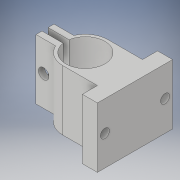
# Autodesk Inventor part: round_adaptor_13
Saved by Autodesk Inventor 2019 (Build 230136000, 136)
## iProperties
Created: 2018-09-01
Part Number: round_adaptor_13
Material: Generic
Document SubType Name: Modeling
Designer: cruiser
Density: 1 g/cm^3
Appearance: Default
Author: cruiser
Autodesk Inventor part; units mm, degrees
ref_plane "YZ Plane" through (0, 0, 0) normal (1, 0, 0) x (0, 1, 0)
ref_plane "XZ Plane" through (0, 0, 0) normal (0, 1, 0) x (-1, 0, 0)
ref_plane "XY Plane" through (0, 0, 0) normal (0, 0, 1) x (1, 0, 0)
sketch "Sketch1" plane through (0, 0, 0) normal (0, 1, 0) x (-1, 0, 0)
  arc A0 (0, 6.5) -> (0, -6.5) centre (0, 0) ccw
  arc A1 (7.433, 1) -> (6.8739, 3) centre (0, 0) ccw
  line L0 (0, 7.5) -> (-16.5, 7.5)
  line L1 (-16.5, 7.5) -> (-16.5, -7.5)
  line L2 (-16.5, -7.5) -> (0, -7.5)
  line L3 (0, -7.5) -> (0, -6.5)
  line L4 (-16.5, 12.5) -> (-11.5, 12.5)
  line L5 (-11.5, 12.5) -> (-11.5, 7.5)
  line L6 (-11.5, 7.5) -> (-16.5, 7.5)
  line L7 (-16.5, 7.5) -> (-16.5, 12.5)
  line L8 (-16.5, -7.5) -> (-11.5, -7.5)
  line L9 (-11.5, -7.5) -> (-11.5, -12.5)
  line L10 (-11.5, -12.5) -> (-16.5, -12.5)
  line L11 (-16.5, -12.5) -> (-16.5, -7.5)
  line L12 (6.4226, 1) -> (13.4226, 1)
  line L13 (13.4226, 1) -> (13.4226, 3)
  line L14 (13.4226, 3) -> (6.4226, 3)
  line L15 (6.4226, 3) -> (6.4226, 1)
  line L16 (0, 0) -> (-6.5, 0)
  line L17 (6.4226, -1) -> (13.4226, -1)
  line L18 (13.4226, -1) -> (13.4226, -3)
  line L19 (13.4226, -3) -> (6.4226, -3)
  line L20 (6.4226, -3) -> (6.4226, -1)
  arc A2 (7.433, -1) -> (7.5, 0) centre (0, 0) ccw
  arc A3 (6.8739, 3) -> (6.8739, -3) centre (0, 0) ccw
  arc A4 (6.4226, 1) -> (0, 6.5) centre (0, 0) ccw
  arc A5 (7.5, 0) -> (7.433, 1) centre (0, 0) ccw
  arc A6 (6.4226, -1) -> (6.5, 0) centre (0, 0) ccw
  arc A7 (6.8739, -3) -> (7.433, -1) centre (0, 0) ccw
  arc A8 (0, -6.5) -> (5.7663, -3) centre (0, 0) ccw
  line L21 (0, -6.5) -> (0, 6.5)
  line L22 (0, 6.5) -> (0, 7.5)
  arc A9 (5.7663, -3) -> (6.4226, -1) centre (0, 0) ccw
  arc A10 (6.5, 0) -> (6.4226, 1) centre (0, 0) ccw
  dimension "d0" = 13
  dimension "d1" = 15
  dimension "d2" = 15
  dimension "d3" = 16.5
  dimension "d4" = 5
  dimension "d5" = 5
  dimension "d6" = 5
  dimension "d7" = 5
  dimension "d8" = 1
  dimension "d9" = 2
  dimension "d10" = 7
  constraints: 46 end point, 31 point on circle, 11 centre point, 10 parallel, 9 point on line, 5 horizontal, 4 perpendicular, 4 symmetric about line, 2 coincident, 1 collinear
  measures "d0" diameter of A0
  measures "d1" diameter of A1
  measures "d2" distance of L2.end L0.start
  measures "d3" distance of L0.start L0.end
  measures "d4" distance of L4.start L4.end
  measures "d5" distance of L8.end L9.end
  measures "d6" distance of L9.end L10.end
  measures "d7" distance of L4.end L5.end
  measures "d8" distance between parallel lines of L16 L12
  measures "d9" distance of L12.end L13.end
  measures "d10" distance of L13.end L14.end
extrude "Extrusion1" add sketch "Sketch1" along normal blind 20 contours L22 A3 L14 L15 A4 | A0 L3 A3 L22 | L15 L14 A1 L12 | A3 L2 L1 L0 | A8 A9 L20 L19 A3 L3 | A1 L14 L13 L12 | L0 L7 L4 L5 | L17 A7 L19 L20 | L9 L10 L11 L2 | A7 L17 L18 L19
sketch "Sketch2" plane through (16.5, 0, 12.5) normal (1, 0, 0) x (0, 0, -1)
  circle A0 centre (22.5, 10) radius 1.5
  line L0 (12.5, 0) -> (12.5, 20)
  line L1 (11.5, 0) -> (11.5, 20) projected
  line L2 (0, 0) -> (25, 0) projected
  circle A1 centre (2.5, 10) radius 1.5
  dimension "d13" = 3
  dimension "d14" = 10
  dimension "d15" = 10
  constraints: 2 centre point, 2 end point, 1 parallel, 1 symmetric about line, 1 other
  measures "d13" diameter of A0
  measures "d14" distance from line of L2 A0.centre
  measures "d15" distance from line of L0 A0.centre
extrude "Extrusion2" cut sketch "Sketch2" against normal up to next
sketch "Sketch3" plane through (-13.4226, 0, 3) normal (0, 0, 1) x (1, 0, 0)
  circle A0 centre (2.5488, 10) radius 1.75
  line L0 (6.5488, 20) -> (6.5488, 0) projected
  line L1 (0, 0) -> (6.5488, 0) projected
  point P0 (13.4226, 0)
  dimension "d18" = 4
  dimension "d19" = 3.5
  dimension "d20" = 10
  constraints: 1 centre point
  measures "d18" distance from line of L0 A0.centre
  measures "d19" diameter of A0
  measures "d20" distance from line of L1 A0.centre
extrude "Extrusion3" cut sketch "Sketch3" against normal up to next
sketch "Sketch4" plane through (-6.8739, 0, -3) normal (0, 0, -1) x (-1, 0, 0)
  circle A0 centre (4, 10) radius 1.5
  line L0 (0, 0) -> (0, 20) projected
  line L1 (0, 0) -> (6.5488, 0) projected
  point P0 (-6.8739, 0)
  dimension "d23" = 4
  dimension "d24" = 10
  dimension "d25" = 3
  constraints: 1 centre point
  measures "d23" distance from line of L0 A0.centre
  measures "d24" distance from line of L1 A0.centre
  measures "d25" diameter of A0
extrude "Extrusion4" cut sketch "Sketch4" against normal up to next
body "Solid1"
